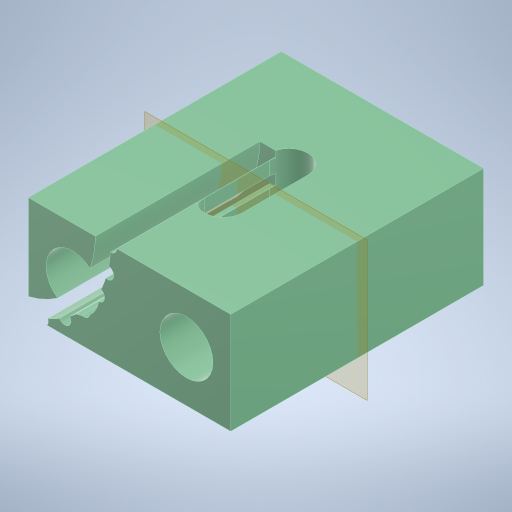
# Autodesk Inventor part: стена_каретки
Saved by Autodesk Inventor 2023.1 (Build 271208000, 208)
## iProperties
Created: 2026-01-04
Part Number: стена_каретки
Material: Полипропилен
Document SubType Name: Modeling
Designer: DELL
Density: 0.899 g/cm^3
Appearance: Гладкий — темный цвет морской волны
Author: DELL
Autodesk Inventor part; units mm, degrees
ref_plane "YZ Plane" through (0, 0, 0) normal (1, 0, 0) x (0, 1, 0)
ref_plane "XZ Plane" through (0, 0, 0) normal (0, 1, 0) x (-1, 0, 0)
sketch "Эскиз1" plane through (0, 0, 0) normal (0, 0, 1) x (1, 0, 0)
  line L0 (13.5, 19.05) -> (-13.5, 19.05) construction
  circle A0 centre (-7.5, -8) radius 1.6 construction
  circle A1 centre (7.5, -8) radius 1.6 construction
  line L1 (-13.5, 19.05) -> (2.5, 19.05)
  line L2 (-13.5, 19.05) -> (-13.5, 9.05)
  line L3 (-13.5, 11.05) -> (2.5, 11.05)
  line L4 (-13.5, 11.05) -> (-13.5, 9.05)
  line L5 (2.5, 11.05) -> (2.5, 19.05)
  point P0 (2.5, 15.05)
  dimension "d3" = 0
  dimension "d15" = 16
  constraints: 10 end point, 1 collinear, 1 midpoint, 1 parallel, 1 vertical
  measures "d3" distance from line of L3.start L2
  measures "d15" distance from line of L2 point (2.5, 15.05)
extrude "Выдавливание1" add sketch "Эскиз1" along normal blind 20
ref_plane "РабПлоскость1" through (0, 0, 10) normal (0, 0, -1) x (-1, 0, 0)
sketch "Эскиз4" plane through (0, 0, 20) normal (0, 0, 1) x (1, 0, 0)
  line L0 (2.5, 11.05) -> (2.5, 19.05) construction
  line L1 (2.5, 15.05) -> (-13.5, 15.05) construction
  line L2 (-13.5, 19.05) -> (-13.5, 11.05) construction
  circle A0 centre (-10, 15.05) radius 2.1
  circle A1 centre (-1, 15.05) radius 2.1
  point P0 (0, 0)
  point P1 (-13.5, 9.05)
  dimension "d16" = 4.2
  dimension "d17" = 4.2
  dimension "d18" = 3.5
  dimension "d19" = 3.5
  constraints: 2 centre point, 2 end point, 2 midpoint, 2 point on line, 1 horizontal
  measures "d16" diameter of A0
  measures "d17" diameter of A1
  measures "d18" distance from line of L0 A1.centre
  measures "d19" distance from line of L2 A0.centre
extrude "Выдавливание4" cut sketch "Эскиз4" against normal blind 5
mirror "Зеркальное отражение2" about plane through (0, 0, 10) normal (0, 0, -1) of "Выдавливание4"
sketch "Эскиз5" plane through (-13.5, 19.05, 0) normal (0, 1, 0) x (1, 0, 0)
  line L0 (16, 0) -> (0, 0) construction
  line L1 (0, 0) -> (0, -20) construction
  line L2 (16, -20) -> (0, -20) construction
  line L3 (16, 0) -> (16, -20) construction
  line L4 (8, -7.407) -> (8, -12.593) construction
  line L5 (6.5, -7.407) -> (6.5, -12.593)
  line L6 (9.5, -12.593) -> (9.5, -7.407)
  arc A0 (9.5, -7.407) -> (6.5, -7.407) centre (8, -7.407) ccw
  arc A1 (6.5, -12.593) -> (9.5, -12.593) centre (8, -12.593) ccw
  point P0 (13.5, 0)
  point P1 (8, -10)
  dimension "d22" = 3
  constraints: 8 end point, 4 point on circle, 4 tangent, 2 centre point, 1 midpoint, 1 parallel, 1 vertical
  measures "d22" diameter of A1
extrude "Выдавливание5" cut sketch "Эскиз5" against normal blind 20
ref_plane "РабПлоскость2" through (0, 0, 10) normal (0, 0, 1) x (1, 0, 0)
sketch "Эскиз7" plane through (0, 0, 10) normal (0, 0, 1) x (1, 0, 0)
  line L0 (-7, 19.05) -> (-7, 11.05) construction
  arc A0 (-13.5, 11.05) -> (-12.8908, 11.202) centre (-15.1731, 19.05) ccw
  arc A1 (-7, 19.55) -> (-7.0153, 18.5502) centre (-7, 19.05) ccw construction
  line L1 (-7, 19.05) -> (-7, 19.55) construction
  arc A2 (-7, 16.629) -> (-7.1382, 17.5535) centre (-7.2447, 17.065) ccw
  arc A3 (-7.7422, 15.6469) -> (-8.2131, 14.7653) centre (-7.9642, 15.1989) ccw construction
  arc A4 (-8.7912, 13.9441) -> (-9.4621, 13.2033) centre (-9.1153, 13.5634) ccw construction
  arc A5 (-10.2223, 12.547) -> (-11.0531, 11.9913) centre (-10.6292, 12.2564) ccw construction
  arc A6 (-11.9499, 11.5393) -> (-12.8908, 11.202) centre (-12.4152, 11.3563) ccw construction
  arc A7 (-7, 18.55) -> (-6.5, 19.05) centre (-7, 19.05) ccw
  arc A8 (-7.3809, 16.5839) -> (-7, 16.629) centre (-7.2447, 17.065) ccw
  arc A9 (-7.1382, 17.5535) -> (-7.3809, 16.5839) centre (-7.2447, 17.065) ccw construction
  arc A10 (-8.2131, 14.7653) -> (-7.7422, 15.6469) centre (-7.9642, 15.1989) ccw
  arc A11 (-9.4621, 13.2033) -> (-8.7912, 13.9441) centre (-9.1153, 13.5634) ccw
  arc A12 (-11.0531, 11.9913) -> (-10.2223, 12.547) centre (-10.6292, 12.2564) ccw
  arc A13 (-12.8908, 11.202) -> (-11.9499, 11.5393) centre (-12.4152, 11.3563) ccw
  line L2 (-4, 11.05) -> (-7, 11.05) projected
  arc A14 (-7.0153, 18.5502) -> (-7, 19.05) centre (-15.1731, 19.05) ccw construction
  arc A15 (-7.1382, 17.5535) -> (-7.0153, 18.5502) centre (-15.1731, 19.05) ccw
  arc A16 (-7.7422, 15.6469) -> (-7.3809, 16.5839) centre (-15.1731, 19.05) ccw
  arc A17 (-7.3809, 16.5839) -> (-7.1382, 17.5535) centre (-15.1731, 19.05) ccw construction
  arc A18 (-8.2131, 14.7653) -> (-7.7422, 15.6469) centre (-15.1731, 19.05) ccw construction
  arc A19 (-8.7912, 13.9441) -> (-8.2131, 14.7653) centre (-15.1731, 19.05) ccw
  arc A20 (-9.4621, 13.2033) -> (-8.7912, 13.9441) centre (-15.1731, 19.05) ccw construction
  arc A21 (-11.0531, 11.9913) -> (-10.2223, 12.547) centre (-15.1731, 19.05) ccw construction
  arc A22 (-11.9499, 11.5393) -> (-11.0531, 11.9913) centre (-15.1731, 19.05) ccw
  arc A23 (-12.8908, 11.202) -> (-11.9499, 11.5393) centre (-15.1731, 19.05) ccw construction
  arc A24 (-10.2223, 12.547) -> (-9.4621, 13.2033) centre (-15.1731, 19.05) ccw
  arc A25 (-13.5, 12.2806) -> (-8.2, 19.05) centre (-15.1731, 19.05) ccw
  line L3 (-8.2, 19.05) -> (-6.5, 19.05)
  line L4 (2.5, 19.05) -> (-13.5, 19.05) projected
  line L5 (-13.5, 19.05) -> (-13.5, 11.05) projected
  line L6 (-13.5, 11.05) -> (-13.5, 12.2806)
  arc A26 (-7.0153, 18.5502) -> (-7, 18.55) centre (-7, 19.05) ccw
  line L7 (-13.5, 11.05) -> (-12.4152, 10.8563)
  point P0 (0, 0)
  point P1 (-7, 19.05)
  point P2 (-7.0153, 18.5502)
  dimension "d25" = 1
  dimension "d34" = 1
  dimension "d36" = 1
  dimension "d39" = 1
  dimension "d40" = 1
  dimension "d41" = 1
  dimension "d42" = 1
  dimension "d43" = 1
  dimension "d44" = 1
  dimension "d45" = 1
  dimension "d46" = 1
  dimension "d48" = 1.2
  constraints: 50 point on circle, 20 centre point, 8 end point, 3 point on line, 2 collinear, 2 vertical, 1 coincident, 101 other
  measures "d25" diameter of A1
  measures "d34" diameter of A2
  measures "d36" diameter of A3
  measures "d41" diameter of A4
  measures "d42" diameter of A5
  measures "d45" diameter of A6
extrude "Выдавливание6" cut sketch "Эскиз7" along normal blind 12 and the other way blind 3 contours L5 A25 L3 A7 A26 A15 A2 A8 A16 A10 A19 A11 A24 A12 A22 A13 L7 A0 | A0 A13 L7
